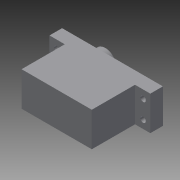
# Autodesk Inventor part: servo
Saved by Autodesk Inventor 2013 (Build 170138000, 138)
## iProperties
Created: 2017-01-26
Part Number: servo
Material: Generic
Document SubType Name: Modeling
Designer: Herman de Vries
Density: 1 g/cm^3
Author: Herman de Vries
Autodesk Inventor part; units mm, degrees
ref_plane "YZ Plane" through (0, 0, 0) normal (1, 0, 0) x (0, 1, 0)
ref_plane "XZ Plane" through (0, 0, 0) normal (0, 1, 0) x (-1, 0, 0)
ref_plane "XY Plane" through (0, 0, 0) normal (0, 0, 1) x (1, 0, 0)
sketch "Sketch1" plane through (0, 0, 0) normal (0, 0, 1) x (1, 0, 0)
  line L0 (0, 0) -> (39, 0)
  line L1 (39, 0) -> (39, 24)
  line L2 (39, 24) -> (0, 24)
  line L3 (0, 24) -> (0, 0)
  line L4 (-8.5, 24) -> (47.5, 24)
  line L5 (47.5, 24) -> (47.5, 31)
  line L6 (47.5, 31) -> (-8.5, 31)
  line L7 (-8.5, 31) -> (-8.5, 24)
  point P0 (19.5, 24)
  dimension "d0" = 39
  dimension "d1" = 24
  dimension "d2" = 56
  dimension "d3" = 7
  constraints: 16 end point, 4 parallel, 2 horizontal, 2 midpoint, 2 perpendicular, 1 coincident
  measures "d0" distance of L2.end L1.end
  measures "d1" distance of L1.end L0.end
  measures "d2" distance of L5.end L6.end
  measures "d3" distance of L6.end L4.start
extrude "Extrusion1" add sketch "Sketch1" along normal blind 19
sketch "Sketch2" plane through (-8.5, 31, 0) normal (0, 1, 0) x (1, 0, 0)
  circle A0 centre (18, -9.5) radius 6
  line L0 (0, 0) -> (0, -19) projected
  circle A1 centre (18, -9.5) radius 1.5
  point P0 (8.5, 0)
  point P1 (0, -9.5)
  dimension "d6" = 12
  dimension "d7" = 18
  dimension "d8" = 3
  constraints: 2 centre point, 1 coincident, 1 horizontal alignment, 1 midpoint
  measures "d6" diameter of A0
  measures "d7" distance from line of A0.centre L0
  measures "d8" diameter of A1
extrude "Extrusion2" add sketch "Sketch2" along normal blind 6
sketch "Sketch3" plane through (-8.5, 31, 0) normal (0, 1, 0) x (1, 0, 0)
  line L0 (4, -4.5) -> (52, -4.5) construction
  line L1 (52, -4.5) -> (52, -14.5) construction
  line L2 (52, -14.5) -> (4, -14.5) construction
  line L3 (4, -14.5) -> (4, -4.5) construction
  circle A0 centre (4, -4.5) radius 1.5
  circle A1 centre (4, -14.5) radius 1.5
  circle A2 centre (52, -14.5) radius 1.5
  circle A3 centre (52, -4.5) radius 1.5
  line L4 (0, 0) -> (0, -19) projected
  line L5 (56, 0) -> (56, -19) projected
  point P0 (8.5, 0)
  dimension "d11" = 3
  dimension "d12" = 3
  dimension "d13" = 3
  dimension "d14" = 3
  dimension "d15" = 4
  dimension "d16" = 4
  dimension "d17" = 4.5
  dimension "d18" = 4.5
  constraints: 8 end point, 4 centre point, 4 coincident, 2 parallel, 1 horizontal, 1 perpendicular
  measures "d11" diameter of A0
  measures "d12" diameter of A1
  measures "d13" diameter of A2
  measures "d14" diameter of A3
  measures "d15" distance between parallel lines of L4 L3
  measures "d16" distance between parallel lines of L1 L5
  measures "d17" distance from line of L4.start L0
  measures "d18" vertical distance of L4.end L2.end
extrude "Extrusion3" cut sketch "Sketch3" against normal blind 10
body "Solid1"
